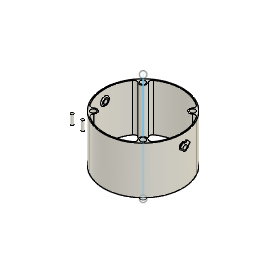
Middle_Section_v4 (Autodesk Fusion 360 design; units mm, degrees)
part number: 2025-04-25-07-19-05-097
part number: 2025-04-25-07-19-30-780
Autodesk Fusion 360 part; units mm, degrees
note: some values were not read from the file. Chosen so that the rebuilt part matches the saved one: which face or edge a step refers to. Set by a fixed rule: which sketch regions a step uses.
sketch "Sketch1" plane through (0, 0, 0) normal (0, 0, 1) x (1, 0, 0) in component "Middle"
  circle A0 centre (0, 0) radius 75
  dimension "d1" = 150
  constraint coincident A0.centre origin
  measures "d1" diameter of A0
extrude "Extrude1" add sketch "Sketch1" along normal blind 90 makes body 1 in component "Middle"
shell "Shell1" thickness 2 removed faces 2 at (17.7838, -26.6668, 90) at (17.7838, -26.6668, 0) on bodies 1 in component "Middle"
ref_plane "WorkPlane1" through (-71, 0, 0) normal (1, 0, 0) x (0, 1, 0) in component "Middle"
sketch "Sketch2" plane through (-71, 0, 0) normal (1, 0, 0) x (0, 1, 0) in component "Middle"
  circle A0 centre (0, 70) radius 6
  dimension "d6" = 12
  measures "d6" diameter of A0
extrude "Extrude2" add sketch "Sketch2" against normal blind 9 bodies 1 in component "Middle"
sketch "Sketch10" plane through (-80, 0, 0) normal (-1, 0, 0) x (0, -1, 0) in component "Middle"
  circle A0 centre (0, 70) radius 6
  arc A1 (10, 70) -> (-10, 70) centre (0, 70) ccw
  line L0 (-10, 70) -> (10, 70)
  constraint coincident A0.centre A1.centre
  constraint horizontal L0
extrude "Extrude9" add sketch "Sketch10" against normal blind 2 contours A0 A1 L0 bodies 1 in component "Middle"
sketch "Sketch12" plane through (-80, 0, 0) normal (-1, 0, 0) x (0, -1, 0) in component "Middle"
  arc A0 (-6, 70) -> (6, 70) centre (0, 70) ccw
  line L0 (6, 70) -> (10, 70)
  arc A1 (10, 70) -> (-10, 70) centre (0, 70) ccw
  line L1 (-10, 70) -> (-6, 70)
  circle A2 centre (0, 70) radius 4
  dimension "d59" = 8
  constraint concentric A0 A2
  measures "d59" diameter of A2
extrude "Extrude11" cut sketch "Sketch12" against normal blind 10 contours A2 bodies 1 in component "Middle"
sketch "Sketch13" plane through (-80, 0, 0) normal (-1, 0, 0) x (0, -1, 0) in component "Middle"
  circle A0 centre (0, 70) radius 4
  arc A1 (-6, 70) -> (6, 70) centre (0, 70) ccw
  line L0 (6, 70) -> (10, 70)
  arc A2 (10, 70) -> (-10, 70) centre (0, 70) ccw
  line L1 (-10, 70) -> (-6, 70)
  circle A3 centre (0, 80) radius 2.8
  dimension "d62" = 5.6
  constraint midpoint A2 A3.centre
  measures "d62" diameter of A3
extrude "Extrude12" cut sketch "Sketch13" against normal blind 2 contours A2 A3 | A2 A3 bodies 1 in component "Middle"
sketch "Sketch5" plane through (0, 0, 0) normal (0, 1, 0) x (1, 0, 0) in component "Middle"
  line L0 (0, 54.8049) -> (0, -150)
  constraint vertical L0
sketch "Sketch6" plane through (0, 0, 0) normal (0, 0, 1) x (1, 0, 0) in component "Middle"
  line L0 (-75, -75) -> (75, 75) construction
  line L1 (-75, 75) -> (75, -75) construction
  circle A0 centre (0, 0) radius 74
  circle A1 centre (-52.3259, -52.3259) radius 7 construction
  circle A2 centre (-52.3259, 52.3259) radius 7 construction
  circle A3 centre (52.3259, 52.3259) radius 7 construction
  circle A4 centre (52.3259, -52.3259) radius 7 construction
  circle A5 centre (-47.3762, -47.3762) radius 7
  circle A6 centre (-47.3762, 47.3762) radius 7
  circle A7 centre (47.3762, 47.3762) radius 7
  circle A8 centre (47.3762, -47.3762) radius 7
  dimension "d19" = 14
  dimension "d20" = 14
  dimension "d21" = 14
  dimension "d22" = 14
  constraint perpendicular L0 L1
  constraint coincident A0.centre origin
  constraint coincident A0 A1.centre
  constraint coincident L0 A1.centre
  constraint coincident L1 A2.centre
  constraint coincident A0 A2.centre
  constraint coincident A0 A3.centre
  constraint coincident L0 A3.centre
  constraint coincident A0 A4.centre
  constraint coincident L1 A4.centre
  constraint coincident L0 A5.centre
  constraint coincident A1 A5.centre
  constraint coincident A1.centre A5
  constraint tangent A0 A5
  constraint coincident A2 A6.centre
  constraint coincident L1 A6.centre
  constraint coincident A2.centre A6
  constraint tangent A0 A6
  constraint coincident A3 A7.centre
  constraint coincident L0 A7.centre
  constraint coincident A3.centre A7
  constraint coincident A4 A8.centre
  constraint coincident L1 A8.centre
  constraint coincident A4.centre A8
  measures "d19" diameter of A1
  measures "d20" diameter of A2
  measures "d21" diameter of A3
  measures "d22" diameter of A4
extrude "Extrude5" add sketch "Sketch6" along normal blind 90 contours A7 | A6 | A5 | A8 bodies 1 in component "Middle"
sketch "Sketch7" plane through (0, 0, 90) normal (0, 0, 1) x (-1, 0, 0) in component "Middle"
  arc A0 (-48.8899, -54.2105) -> (48.8899, -54.2105) centre (0, 0) ccw
  arc A1 (-48.8899, -54.2105) -> (-54.2105, -48.8899) centre (-47.3762, -47.3762) ccw
  arc A2 (-54.2105, 48.8899) -> (-54.2105, -48.8899) centre (0, 0) ccw
  arc A3 (-54.2105, 48.8899) -> (-48.8899, 54.2105) centre (-47.3762, 47.3762) ccw
  arc A4 (48.8899, 54.2105) -> (-48.8899, 54.2105) centre (0, 0) ccw
  arc A5 (48.8899, 54.2105) -> (54.2105, 48.8899) centre (47.3762, 47.3762) ccw
  arc A6 (54.2105, -48.8899) -> (54.2105, 48.8899) centre (0, 0) ccw
  arc A7 (54.2105, -48.8899) -> (48.8899, -54.2105) centre (47.3762, -47.3762) ccw
  circle A8 centre (0, 0) radius 75
  circle A9 centre (47.3762, 47.3762) radius 5
  circle A10 centre (47.3762, -47.3762) radius 5
  circle A11 centre (-47.3762, -47.3762) radius 5
  circle A12 centre (-47.3762, 47.3762) radius 5
  dimension "d25" = 10
  dimension "d26" = 10
  dimension "d27" = 10
  dimension "d28" = 10
  constraint concentric A5 A9
  constraint concentric A7 A10
  constraint concentric A1 A11
  constraint concentric A3 A12
  measures "d25" diameter of A9
  measures "d26" diameter of A10
  measures "d27" diameter of A11
  measures "d28" diameter of A12
sketch "Sketch8" plane through (0, 0, 0) normal (0, 0, -1) x (1, 0, 0) in component "Middle"
  circle A0 centre (0, 0) radius 75
  arc A1 (-54.2105, 48.8899) -> (-54.2105, -48.8899) centre (0, 0) ccw
  arc A2 (-54.2105, 48.8899) -> (-48.8899, 54.2105) centre (-47.3762, 47.3762) ccw
  arc A3 (48.8899, 54.2105) -> (-48.8899, 54.2105) centre (0, 0) ccw
  arc A4 (48.8899, 54.2105) -> (54.2105, 48.8899) centre (47.3762, 47.3762) ccw
  arc A5 (54.2105, -48.8899) -> (54.2105, 48.8899) centre (0, 0) ccw
  arc A6 (54.2105, -48.8899) -> (48.8899, -54.2105) centre (47.3762, -47.3762) ccw
  arc A7 (-48.8899, -54.2105) -> (48.8899, -54.2105) centre (0, 0) ccw
  arc A8 (-48.8899, -54.2105) -> (-54.2105, -48.8899) centre (-47.3762, -47.3762) ccw
  circle A9 centre (-47.3762, 47.3762) radius 4.7
  circle A10 centre (47.3762, 47.3762) radius 4.7
  circle A11 centre (47.3762, -47.3762) radius 4.7
  circle A12 centre (-47.3762, -47.3762) radius 4.7
  dimension "d29" = 9.4
  dimension "d30" = 9.4
  dimension "d31" = 9.4
  dimension "d32" = 9.4
  constraint concentric A2 A9
  constraint concentric A4 A10
  constraint concentric A6 A11
  constraint concentric A8 A12
  measures "d29" diameter of A9
  measures "d30" diameter of A10
  measures "d31" diameter of A11
  measures "d32" diameter of A12
extrude "Extrude6" add sketch "Sketch8" along normal blind 6 contours A9 | A10 | A11 | A12 bodies 1 in component "Middle"
extrude "Extrude7" cut sketch "Sketch7" against normal blind 8 contours A9 | A10 | A11 | A12 bodies 1 in component "Middle"
fillet "Fillet2" radius 6 8 edges at (54.2105, 48.8899, 45) (48.8899, 54.2105, 45) (48.8899, -54.2105, 45) (54.2105, -48.8899, 45) (-48.8899, -54.2105, 45) (-48.8899, 54.2105, 45) (-54.2105, -48.8899, 45) (-54.2105, 48.8899, 45) on bodies 1 in component "Middle"
sketch "Sketch9" plane through (0, 0, 0) normal (0, 0, 1) x (1, 0, 0) in component "Middle"
  circle A0 centre (-125, 0) radius 2.5
  circle A1 centre (-135, 0) radius 2.5
  dimension "d39" = 5
  dimension "d40" = 5
  measures "d39" diameter of A0
  measures "d40" diameter of A1
extrude "Extrude8" add sketch "Sketch9" along normal blind 20 separate body makes body 2 at (-122.5031, -0.1246, 13.3333) makes body 3 at (-134.3229, 2.4066, 13.3333) in component "Middle"
move_body "Move1" bodies 2 to x (1, 0, 0) y (0, 1, 0) z (0, 0, 1) at (10, 0, 0) in component "Middle"
fillet "Fillet3" radius 2 2 edges at (-117.3308, -0.904, 20) (-137.3308, -0.904, 20) on bodies 2 3 in component "Middle"
mirror "Mirror3" about plane through (0, 0, -6) normal (1, 0, 0) of "Extrude2", "Extrude9", "Extrude11", "Extrude12" in component "Middle"
chamfer "Chamfer2" distance 4 angle 45 4 edges at (79, 10, 70) (79, -10, 70) (-79, -10, 70) (-79, 10, 70) on bodies 1 in component "Middle"
fillet "Fillet5" radius 2 4 edges at (72.8565, 4.5745, 66.1175) (72.753, -6, 70) (72.8565, 4.5745, 73.8825) (-72.753, -6, 69.9968) on bodies 1 in component "Middle"
component "Middle" placed x (1, 0, 0) y (0, 1, 0) z (0, 0, 1) at (0, 0, 6)
